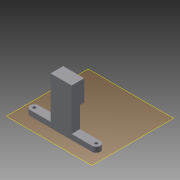
# Autodesk Inventor part: HornBase
Saved by Autodesk Inventor 2014 SP1 (Build 180222100, 222)
## iProperties
Created: 2017-05-14
Part Number: HornBase
Material: Generic
Document SubType Name: Modeling
Designer: danielsikar
Density: 1 g/cm^3
Appearance: Default
Author: danielsikar
Autodesk Inventor part; units mm, degrees
ref_plane "YZ Plane" through (0, 0, 0) normal (1, 0, 0) x (0, 1, 0)
ref_plane "XZ Plane" through (0, 0, 0) normal (0, 1, 0) x (-1, 0, 0)
ref_plane "Work Plane1" through (-43.75, 3, -4) normal (0, 0, 1) x (-1, 0, 0)
sketch "Sketch1" plane through (-43.75, 3, -4) normal (0, 0, 1) x (-1, 0, 0)
  circle A0 centre (-9.7413, 6.5) radius 0.7 projected
  circle A1 centre (19.7413, 6.5) radius 0.7 projected
  circle A2 centre (-9.7413, 6.5) radius 2
  circle A3 centre (19.7413, 6.5) radius 2
  line L0 (-9.7413, 8.5) -> (19.7413, 8.5)
  line L1 (-9.7413, 4.5) -> (19.7413, 4.5)
  point P0 (-43.75, 3)
  dimension "d0" = 4
  dimension "d1" = 4
  constraints: 4 end point, 4 point on circle, 2 centre point, 2 tangent
  measures "d0" diameter of A2
  measures "d1" diameter of A3
extrude "Extrusion1" add sketch "Sketch1" along normal blind 2.5
sketch "Sketch2" plane through (-43.75, 3, -1.5) normal (0, 0, 1) x (1, 0, 0)
  line L0 (9.7413, -4.5) -> (-19.7413, -4.5) projected
  line L1 (-19.7413, -8.5) -> (9.7413, -8.5) projected
  line L2 (-10, -4.5) -> (0, -4.5)
  line L3 (0, -4.5) -> (0, -8.5)
  line L4 (0, -8.5) -> (-10, -8.5)
  line L5 (-10, -8.5) -> (-10, -4.5)
  circle A0 centre (-5, -6.5) radius 1.25 projected
  point P0 (43.75, -3)
  dimension "d4" = 10
  dimension "d6" = 5
  constraints: 8 end point, 2 parallel, 2 point on line, 1 horizontal, 1 perpendicular
  measures "d4" distance of L3.end L4.end
  measures "d6" distance from line of L3 A0.centre
extrude "Extrusion2" add sketch "Sketch2" along normal blind 20 contours L3 L1 L5 L0 | A0
sketch "Sketch3" plane through (-63.4913, -1.5, -4) normal (0, 1, 0) x (1, 0, 0)
  line L0 (19.7413, -2.5) -> (19.7413, -22.5) projected
  line L1 (9.7413, -22.5) -> (19.7413, -22.5)
  line L2 (19.7413, -22.5) -> (19.7413, -12.5)
  line L3 (19.7413, -12.5) -> (9.7413, -12.5)
  line L4 (9.7413, -12.5) -> (9.7413, -22.5)
  point P0 (63.4913, -4)
  constraints: 8 end point, 2 parallel, 1 horizontal, 1 midpoint, 1 perpendicular
extrude "Extrusion3" add sketch "Sketch3" along normal blind 1.5
fillet "Fillet1" radius 2 2 edges at (-53.75, -2.75, 18.5) (-43.75, -2.75, 18.5)
body "Solid1"
